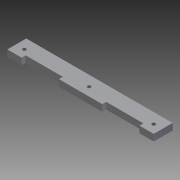
# Autodesk Inventor part: carro x lado polea pieza3
Saved by Autodesk Inventor 2012 (Build 160160000, 160)
## iProperties
Created: 2014-12-17
Part Number: carro x lado polea pieza3
Material: Default
Document SubType Name: Modeling
Designer: PRINCIPAL
Density: 1 g/cm^3
Author: PRINCIPAL
Autodesk Inventor part; units mm, degrees
ref_plane "YZ Plane" through (0, 0, 0) normal (1, 0, 0) x (0, 1, 0)
ref_plane "XZ Plane" through (0, 0, 0) normal (0, 1, 0) x (-1, 0, 0)
ref_plane "XY Plane" through (0, 0, 0) normal (0, 0, 1) x (1, 0, 0)
sketch "Boceto1" plane through (0, 0, 0) normal (0, 0, 1) x (1, 0, 0)
  arc A0 (4.65, 21.5) -> (6, 20.15) centre (6, 21.5) ccw
  arc A1 (6, 20.15) -> (7.35, 21.5) centre (6, 21.5) ccw
  arc A2 (7.35, 21.5) -> (6, 22.85) centre (6, 21.5) ccw
  arc A3 (6, 22.85) -> (4.65, 21.5) centre (6, 21.5) ccw
  arc A4 (53.65, 21.5) -> (55, 20.15) centre (55, 21.5) ccw
  arc A5 (55, 20.15) -> (56.35, 21.5) centre (55, 21.5) ccw
  arc A6 (56.35, 21.5) -> (55, 22.85) centre (55, 21.5) ccw
  arc A7 (55, 22.85) -> (53.65, 21.5) centre (55, 21.5) ccw
  arc A8 (104, 22.8571) -> (102.6429, 21.5) centre (104, 21.5) ccw
  arc A9 (102.6429, 21.5) -> (104, 20.1429) centre (104, 21.5) ccw
  arc A10 (104, 20.1429) -> (105.3571, 21.5) centre (104, 21.5) ccw
  arc A11 (105.3571, 21.5) -> (104, 22.8571) centre (104, 21.5) ccw
  line L0 (-0.4, 15.1) -> (-0.4, 29.4)
  line L1 (-0.4, 29.4) -> (110.4, 29.4)
  line L2 (110.4, 29.4) -> (110.4, 15.1)
  line L3 (110.4, 15.1) -> (99.6, 15.1)
  line L4 (99.6, 15.1) -> (99.6, 18.1)
  line L5 (99.6, 18.1) -> (71.4, 18.1)
  line L6 (71.4, 18.1) -> (71.4, 15.1)
  line L7 (71.4, 15.1) -> (38.6, 15.1)
  line L8 (38.6, 15.1) -> (38.6, 18.1)
  line L9 (38.6, 18.1) -> (10.4, 18.1)
  line L10 (10.4, 18.1) -> (10.4, 15.1)
  line L11 (10.4, 15.1) -> (-0.4, 15.1)
  point P0 (0, 0)
  constraints: 24 end point, 24 point on circle, 12 centre point
extrude "Extrusión1" add sketch "Boceto1" along normal blind 5
